Autodesk Fusion 360 part; units mm, degrees
note: some values were not read from the file. Set by a fixed rule: which sketch regions a step uses.
(part 3 of 59)
  spline S10 degree 5 poles (-22.9448, 30.3091) (-22.9448, 30.3092) (-22.945, 30.3093) (-22.9453, 30.3095) (-22.9457, 30.3098) (-22.9463, 30.3103) (-22.9469, 30.3108) (-22.9477, 30.3114) (-22.9486, 30.312) (-22.9496, 30.3127) (-22.9506, 30.3135) (-22.9518, 30.3144) (-22.953, 30.3153) (-22.9543, 30.3162) (-22.9557, 30.3172) (-22.9572, 30.3183) (-22.9588, 30.3195) (-22.9604, 30.3207) (-22.9622, 30.3219) (-22.964, 30.3232) (-22.9659, 30.3246) (-22.9679, 30.326) (-22.9699, 30.3274) (-22.9721, 30.3289) (-22.9743, 30.3305) (-22.9766, 30.3321) (-22.979, 30.3337) (-22.9814, 30.3354) (-22.984, 30.3372) (-22.9866, 30.3389) (-22.9893, 30.3408) (-22.992, 30.3427) (-22.9948, 30.3446) (-22.9978, 30.3465) (-23.0007, 30.3485) (-23.0038, 30.3506) (-23.0069, 30.3527) (-23.0101, 30.3548) (-23.0134, 30.357) (-23.0167, 30.3592) (-23.0201, 30.3614) (-23.0236, 30.3637) (-23.0271, 30.366) (-23.0308, 30.3683) (-23.0344, 30.3707) (-23.0382, 30.3731) (-23.042, 30.3756) (-23.0459, 30.3781) (-23.0499, 30.3806) (-23.0539, 30.3831) (-23.058, 30.3857) (-23.0621, 30.3883) (-23.0664, 30.391) (-23.0706, 30.3937) (-23.075, 30.3964) (-23.0794, 30.3991) (-23.0839, 30.4019) (-23.0884, 30.4047) (-23.093, 30.4075) (-23.0977, 30.4103) (-23.1024, 30.4132) (-23.1072, 30.4161) (-23.1121, 30.4191) (-23.117, 30.422) (-23.122, 30.425) (-23.127, 30.428) (-23.1321, 30.431) (-23.1373, 30.4341) (-23.1425, 30.4372) (-23.1478, 30.4403) (-23.1531, 30.4434) (-23.1585, 30.4466) (-23.164, 30.4497) (-23.1695, 30.4529) (-23.1751, 30.4562) (-23.1807, 30.4594) (-23.1864, 30.4627) (-23.1921, 30.4659) (-23.1979, 30.4692) (-23.2038, 30.4726) (-23.2097, 30.4759) (-23.2157, 30.4793) (-23.2217, 30.4826) (-23.2278, 30.486) (-23.234, 30.4895) (-23.2402, 30.4929) (-23.2464, 30.4963) (-23.2527, 30.4998) (-23.2591, 30.5033) (-23.2655, 30.5068) (-23.272, 30.5103) (-23.2785, 30.5139) (-23.2851, 30.5174) (-23.2918, 30.521) (-23.2984, 30.5246) (-23.3052, 30.5282) (-23.312, 30.5318) (-23.3188, 30.5354) (-23.3257, 30.539) (-23.3327, 30.5427) (-23.3397, 30.5464) (-23.3468, 30.5501) (-23.3539, 30.5538) (-23.361, 30.5575) (-23.3683, 30.5612) (-23.3755, 30.5649) (-23.3828, 30.5687) (-23.3902, 30.5724) (-23.3976, 30.5762) (-23.4051, 30.58) (-23.4126, 30.5838) (-23.4202, 30.5876) (-23.4278, 30.5914) (-23.4355, 30.5952) (-23.4432, 30.5991) (-23.451, 30.6029) (-23.4588, 30.6068) (-23.4666, 30.6106) (-23.4746, 30.6145) (-23.4825, 30.6184) (-23.4905, 30.6223) (-23.4986, 30.6262) (-23.5067, 30.6301) (-23.5149, 30.634) (-23.5231, 30.6379) (-23.5313, 30.6419) (-23.5396, 30.6458) (-23.548, 30.6498) (-23.5564, 30.6537) (-23.5648, 30.6577) (-23.5733, 30.6617) (-23.5818, 30.6657) (-23.5904, 30.6696) (-23.5991, 30.6736) (-23.6077, 30.6776) (-23.6165, 30.6816) (-23.6252, 30.6857) (-23.634, 30.6897) (-23.6429, 30.6937) (-23.6518, 30.6977) (-23.6607, 30.7018) (-23.6697, 30.7058) (-23.6788, 30.7098) (-23.6879, 30.7139) (-23.697, 30.7179) (-23.7062, 30.722) (-23.7154, 30.726) (-23.7247, 30.7301) (-23.734, 30.7342) (-23.7433, 30.7383) (-23.7527, 30.7423) (-23.7622, 30.7464) (-23.7716, 30.7505) (-23.7812, 30.7546) (-23.7907, 30.7587) (-23.8004, 30.7627) (-23.81, 30.7668) (-23.8197, 30.7709) (-23.8295, 30.775) (-23.8393, 30.7791) (-23.8491, 30.7832) (-23.859, 30.7873) (-23.8689, 30.7914) (-23.8788, 30.7955) (-23.8888, 30.7996) (-23.8989, 30.8038) (-23.909, 30.8079) (-23.9191, 30.812) (-23.9292, 30.8161) (-23.9395, 30.8202) (-23.9497, 30.8243) (-23.96, 30.8284) (-23.9703, 30.8325) (-23.9807, 30.8366) (-23.9911, 30.8408) (-24.0016, 30.8449) (-24.0121, 30.849) (-24.0226, 30.8531) (-24.0332, 30.8572) (-24.0438, 30.8613) (-24.0545, 30.8654) (-24.0652, 30.8695) (-24.0759, 30.8736) (-24.0867, 30.8777) (-24.0975, 30.8818) (-24.1084, 30.8859) (-24.1193, 30.89) (-24.1302, 30.8941) (-24.1412, 30.8982) (-24.1522, 30.9023) (-24.1633, 30.9064) (-24.1744, 30.9105) (-24.1855, 30.9146) (-24.1967, 30.9187) (-24.2079, 30.9228) (-24.2191, 30.9269) (-24.2304, 30.9309) (-24.2417, 30.935) (-24.2531, 30.9391) (-24.2645, 30.9431) (-24.276, 30.9472) (-24.2874, 30.9513) (-24.299, 30.9553) (-24.3105, 30.9594) (-24.3221, 30.9634) (-24.3337, 30.9675) (-24.3454, 30.9715) (-24.3571, 30.9756) (-24.3689, 30.9796) (-24.3806, 30.9836) (-24.3925, 30.9877) (-24.4043, 30.9917) (-24.4162, 30.9957) (-24.4281, 30.9997) (-24.4401, 31.0037) (-24.4521, 31.0077) (-24.4642, 31.0117) (-24.4762, 31.0157) (-24.4884, 31.0197) (-24.5005, 31.0237) (-24.5127, 31.0277) (-24.5249, 31.0316) (-24.5372, 31.0356) (-24.5495, 31.0395) (-24.5618, 31.0435) (-24.5742, 31.0475) (-24.5866, 31.0514) (-24.599, 31.0553) (-24.6115, 31.0593) (-24.624, 31.0632) (-24.6365, 31.0671) (-24.6491, 31.071) (-24.6617, 31.0749) (-24.6744, 31.0788) (-24.6871, 31.0827) (-24.6998, 31.0866) (-24.7125, 31.0905) (-24.7253, 31.0943) (-24.7382, 31.0982) (-24.751, 31.1021) (-24.7639, 31.1059) (-24.7743, 31.109) (-24.782, 31.1113) (-24.7872, 31.1128) (-24.7898, 31.1136) knots 0 0 0 0 0 0 0.00416667 0.00833333 0.0125 0.01666667 0.02083333 0.025 0.02916667 0.03333333 0.0375 0.04166667 0.04583333 0.05 0.05416667 0.05833333 0.0625 0.06666667 0.07083333 0.075 0.07916667 0.08333333 0.0875 0.09166667 0.09583333 0.1 0.10416667 0.10833333 0.1125 0.11666667 0.12083333 0.125 0.12916667 0.13333333 0.1375 0.14166667 0.14583333 0.15 0.15416667 0.15833333 0.1625 0.16666667 0.17083333 0.175 0.17916667 0.18333333 0.1875 0.19166667 0.19583333 0.2 0.20416667 0.20833333 0.2125 0.21666667 0.22083333 0.225 0.22916667 0.23333333 0.2375 0.24166667 0.24583333 0.25 0.25416667 0.25833333 0.2625 0.26666667 0.27083333 0.275 0.27916667 0.28333333 0.2875 0.29166667 0.29583333 0.3 0.30416667 0.30833333 0.3125 0.31666667 0.32083333 0.325 0.32916667 0.33333333 0.3375 0.34166667 0.34583333 0.35 0.35416667 0.35833333 0.3625 0.36666667 0.37083333 0.375 0.37916667 0.38333333 0.3875 0.39166667 0.39583333 0.4 0.40416667 0.40833333 0.4125 0.41666667 0.42083333 0.425 0.42916667 0.43333333 0.4375 0.44166667 0.44583333 0.45 0.45416667 0.45833333 0.4625 0.46666667 0.47083333 0.475 0.47916667 0.48333333 0.4875 0.49166667 0.49583333 0.5 0.50416667 0.50833333 0.5125 0.51666667 0.52083333 0.525 0.52916667 0.53333333 0.5375 0.54166667 0.54583333 0.55 0.55416667 0.55833333 0.5625 0.56666667 0.57083333 0.575 0.57916667 0.58333333 0.5875 0.59166667 0.59583333 0.6 0.60416667 0.60833333 0.6125 0.61666667 0.62083333 0.625 0.62916667 0.63333333 0.6375 0.64166667 0.64583333 0.65 0.65416667 0.65833333 0.6625 0.66666667 0.67083333 0.675 0.67916667 0.68333333 0.6875 0.69166667 0.69583333 0.7 0.70416667 0.70833333 0.7125 0.71666667 0.72083333 0.725 0.72916667 0.73333333 0.7375 0.74166667 0.74583333 0.75 0.75416667 0.75833333 0.7625 0.76666667 0.77083333 0.775 0.77916667 0.78333333 0.7875 0.79166667 0.79583333 0.8 0.80416667 0.80833333 0.8125 0.81666667 0.82083333 0.825 0.82916667 0.83333333 0.8375 0.84166667 0.84583333 0.85 0.85416667 0.85833333 0.8625 0.86666667 0.87083333 0.875 0.87916667 0.88333333 0.8875 0.89166667 0.89583333 0.9 0.90416667 0.90833333 0.9125 0.91666667 0.92083333 0.925 0.92916667 0.93333333 0.9375 0.94166667 0.94583333 0.95 0.95416667 0.95833333 0.9625 0.96666667 0.97083333 0.975 0.97916667 0.98333333 0.9875 0.99166667 0.99583333 1 1 1 1 1 1
  line L45 (-13.578, 37.8417) -> (-13.7171, 38.1012)
  line L46 (-13.7171, 38.1012) -> (-13.7175, 38.1019)
  line L47 (-2.0967, 41.1734) -> (-2.1182, 41.4671)
  spline S11 degree 5 poles (-28.5878, 7.3654) (-28.5879, 7.3653) (-28.5881, 7.3653) (-28.5884, 7.3652) (-28.5889, 7.3651) (-28.5896, 7.365) (-28.5905, 7.3648) (-28.5915, 7.3646) (-28.5925, 7.3644) (-28.5937, 7.3642) (-28.595, 7.3639) (-28.5964, 7.3637) (-28.5979, 7.3633) (-28.5995, 7.363) (-28.6012, 7.3626) (-28.603, 7.3623) (-28.6049, 7.3619) (-28.6069, 7.3614) (-28.6089, 7.361) (-28.6111, 7.3605) (-28.6134, 7.36) (-28.6158, 7.3594) (-28.6182, 7.3589) (-28.6208, 7.3583) (-28.6234, 7.3577) (-28.6262, 7.357) (-28.629, 7.3564) (-28.6319, 7.3557) (-28.6349, 7.355) (-28.6379, 7.3542) (-28.6411, 7.3535) (-28.6443, 7.3527) (-28.6477, 7.3519) (-28.6511, 7.351) (-28.6545, 7.3501) (-28.6581, 7.3492) (-28.6617, 7.3483) (-28.6655, 7.3473) (-28.6693, 7.3464) (-28.6731, 7.3454) (-28.6771, 7.3443) (-28.6811, 7.3433) (-28.6852, 7.3422) (-28.6893, 7.3411) (-28.6936, 7.3399) (-28.6979, 7.3387) (-28.7023, 7.3375) (-28.7067, 7.3363) (-28.7112, 7.3351) (-28.7158, 7.3338) (-28.7205, 7.3325) (-28.7252, 7.3311) (-28.73, 7.3298) (-28.7349, 7.3284) (-28.7398, 7.327) (-28.7448, 7.3255) (-28.7498, 7.324) (-28.7549, 7.3225) (-28.7601, 7.321) (-28.7654, 7.3194) (-28.7707, 7.3178) (-28.776, 7.3162) (-28.7815, 7.3146) (-28.7869, 7.3129) (-28.7925, 7.3112) (-28.7981, 7.3095) (-28.8038, 7.3077) (-28.8095, 7.3059) (-28.8153, 7.3041) (-28.8211, 7.3022) (-28.827, 7.3004) (-28.833, 7.2985) (-28.839, 7.2965) (-28.8451, 7.2946) (-28.8512, 7.2926) (-28.8573, 7.2906) (-28.8636, 7.2885) (-28.8699, 7.2864) (-28.8762, 7.2843) (-28.8826, 7.2822) (-28.889, 7.28) (-28.8955, 7.2778) (-28.9021, 7.2756) (-28.9087, 7.2734) (-28.9153, 7.2711) (-28.922, 7.2688) (-28.9288, 7.2664) (-28.9356, 7.2641) (-28.9424, 7.2617) (-28.9493, 7.2592) (-28.9563, 7.2568) (-28.9633, 7.2543) (-28.9703, 7.2518) (-28.9774, 7.2492) (-28.9846, 7.2467) (-28.9918, 7.2441) (-28.999, 7.2414) (-29.0063, 7.2388) (-29.0136, 7.2361) (-29.021, 7.2334) (-29.0284, 7.2306) (-29.0358, 7.2278) (-29.0433, 7.225) (-29.0509, 7.2222) (-29.0585, 7.2193) (-29.0661, 7.2164) (-29.0738, 7.2135) (-29.0815, 7.2105) (-29.0893, 7.2075) (-29.0971, 7.2045) (-29.105, 7.2014) (-29.1129, 7.1984) (-29.1208, 7.1953) (-29.1288, 7.1921) (-29.1368, 7.1889) (-29.1448, 7.1857) (-29.1529, 7.1825) (-29.1611, 7.1793) (-29.1692, 7.176) (-29.1775, 7.1727) (-29.1857, 7.1693) (-29.194, 7.1659) (-29.2023, 7.1625) (-29.2107, 7.1591) (-29.2191, 7.1556) (-29.2276, 7.1521) (-29.2361, 7.1486) (-29.2446, 7.145) (-29.2531, 7.1414) (-29.2617, 7.1378) (-29.2704, 7.1342) (-29.279, 7.1305) (-29.2878, 7.1268) (-29.2965, 7.123) (-29.3053, 7.1193) (-29.3141, 7.1154) (-29.3229, 7.1116) (-29.3318, 7.1078) (-29.3407, 7.1039) (-29.3497, 7.0999) (-29.3587, 7.096) (-29.3677, 7.092) (-29.3767, 7.088) (-29.3858, 7.0839) (-29.395, 7.0799) (-29.4041, 7.0758) (-29.4133, 7.0716) (-29.4225, 7.0675) (-29.4318, 7.0633) (-29.441, 7.059) (-29.4504, 7.0548) (-29.4597, 7.0505) (-29.4691, 7.0462) (-29.4785, 7.0418) (-29.4879, 7.0375) (-29.4974, 7.033) (-29.5069, 7.0286) (-29.5165, 7.0241) (-29.526, 7.0196) (-29.5356, 7.0151) (-29.5452, 7.0105) (-29.5549, 7.006) (-29.5646, 7.0013) (-29.5743, 6.9967) (-29.584, 6.992) (-29.5938, 6.9873) (-29.6036, 6.9825) (-29.6134, 6.9778) (-29.6233, 6.973) (-29.6332, 6.9681) (-29.6431, 6.9633) (-29.653, 6.9584) (-29.663, 6.9534) (-29.673, 6.9485) (-29.683, 6.9435) (-29.6931, 6.9385) (-29.7032, 6.9334) (-29.7133, 6.9283) (-29.7234, 6.9232) (-29.7336, 6.9181) (-29.7437, 6.9129) (-29.754, 6.9077) (-29.7642, 6.9025) (-29.7745, 6.8972) (-29.7847, 6.8919) (-29.7951, 6.8866) (-29.8054, 6.8812) (-29.8158, 6.8758) (-29.8262, 6.8704) (-29.8366, 6.865) (-29.847, 6.8595) (-29.8575, 6.854) (-29.868, 6.8485) (-29.8785, 6.8429) (-29.889, 6.8373) (-29.8996, 6.8317) (-29.9102, 6.826) (-29.9208, 6.8203) (-29.9314, 6.8146) (-29.9421, 6.8088) (-29.9527, 6.803) (-29.9634, 6.7972) (-29.9742, 6.7914) (-29.9849, 6.7855) (-29.9957, 6.7796) (-30.0065, 6.7737) (-30.0173, 6.7677) (-30.0281, 6.7617) (-30.039, 6.7557) (-30.0499, 6.7496) (-30.0608, 6.7435) (-30.0717, 6.7374) (-30.0826, 6.7312) (-30.0936, 6.7251) (-30.1046, 6.7189) (-30.1156, 6.7126) (-30.1266, 6.7063) (-30.1377, 6.7) (-30.1487, 6.6937) (-30.1598, 6.6873) (-30.1709, 6.6809) (-30.1821, 6.6745) (-30.1932, 6.6681) (-30.2044, 6.6616) (-30.2156, 6.6551) (-30.2268, 6.6485) (-30.238, 6.6419) (-30.2492, 6.6353) (-30.2605, 6.6287) (-30.2718, 6.622) (-30.2831, 6.6153) (-30.2944, 6.6086) (-30.3058, 6.6018) (-30.3171, 6.595) (-30.3285, 6.5882) (-30.3399, 6.5813) (-30.3513, 6.5745) (-30.3628, 6.5675) (-30.3742, 6.5606) (-30.3857, 6.5536) (-30.3972, 6.5466) (-30.4064, 6.541) (-30.4133, 6.5367) (-30.4179, 6.5339) (-30.4202, 6.5325) knots 0 0 0 0 0 0 0.00416667 0.00833333 0.0125 0.01666667 0.02083333 0.025 0.02916667 0.03333333 0.0375 0.04166667 0.04583333 0.05 0.05416667 0.05833333 0.0625 0.06666667 0.07083333 0.075 0.07916667 0.08333333 0.0875 0.09166667 0.09583333 0.1 0.10416667 0.10833333 0.1125 0.11666667 0.12083333 0.125 0.12916667 0.13333333 0.1375 0.14166667 0.14583333 0.15 0.15416667 0.15833333 0.1625 0.16666667 0.17083333 0.175 0.17916667 0.18333333 0.1875 0.19166667 0.19583333 0.2 0.20416667 0.20833333 0.2125 0.21666667 0.22083333 0.225 0.22916667 0.23333333 0.2375 0.24166667 0.24583333 0.25 0.25416667 0.25833333 0.2625 0.26666667 0.27083333 0.275 0.27916667 0.28333333 0.2875 0.29166667 0.29583333 0.3 0.30416667 0.30833333 0.3125 0.31666667 0.32083333 0.325 0.32916667 0.33333333 0.3375 0.34166667 0.34583333 0.35 0.35416667 0.35833333 0.3625 0.36666667 0.37083333 0.375 0.37916667 0.38333333 0.3875 0.39166667 0.39583333 0.4 0.40416667 0.40833333 0.4125 0.41666667 0.42083333 0.425 0.42916667 0.43333333 0.4375 0.44166667 0.44583333 0.45 0.45416667 0.45833333 0.4625 0.46666667 0.47083333 0.475 0.47916667 0.48333333 0.4875 0.49166667 0.49583333 0.5 0.50416667 0.50833333 0.5125 0.51666667 0.52083333 0.525 0.52916667 0.53333333 0.5375 0.54166667 0.54583333 0.55 0.55416667 0.55833333 0.5625 0.56666667 0.57083333 0.575 0.57916667 0.58333333 0.5875 0.59166667 0.59583333 0.6 0.60416667 0.60833333 0.6125 0.61666667 0.62083333 0.625 0.62916667 0.63333333 0.6375 0.64166667 0.64583333 0.65 0.65416667 0.65833333 0.6625 0.66666667 0.67083333 0.675 0.67916667 0.68333333 0.6875 0.69166667 0.69583333 0.7 0.70416667 0.70833333 0.7125 0.71666667 0.72083333 0.725 0.72916667 0.73333333 0.7375 0.74166667 0.74583333 0.75 0.75416667 0.75833333 0.7625 0.76666667 0.77083333 0.775 0.77916667 0.78333333 0.7875 0.79166667 0.79583333 0.8 0.80416667 0.80833333 0.8125 0.81666667 0.82083333 0.825 0.82916667 0.83333333 0.8375 0.84166667 0.84583333 0.85 0.85416667 0.85833333 0.8625 0.86666667 0.87083333 0.875 0.87916667 0.88333333 0.8875 0.89166667 0.89583333 0.9 0.90416667 0.90833333 0.9125 0.91666667 0.92083333 0.925 0.92916667 0.93333333 0.9375 0.94166667 0.94583333 0.95 0.95416667 0.95833333 0.9625 0.96666667 0.97083333 0.975 0.97916667 0.98333333 0.9875 0.99166667 0.99583333 1 1 1 1 1 1
  line L48 (-25.6019, 26.2175) -> (-25.6012, 26.2171)
  spline S12 degree 5 poles (-27.0873, 27.5758) (-27.0855, 27.5737) (-27.082, 27.5696) (-27.0767, 27.5635) (-27.0697, 27.5553) (-27.061, 27.545) (-27.0522, 27.5349) (-27.0435, 27.5247) (-27.0347, 27.5146) (-27.026, 27.5045) (-27.0173, 27.4945) (-27.0086, 27.4845) (-26.9999, 27.4745) (-26.9912, 27.4646) (-26.9825, 27.4547) (-26.9738, 27.4448) (-26.9651, 27.435) (-26.9565, 27.4252) (-26.9478, 27.4154) (-26.9392, 27.4057) (-26.9305, 27.396) (-26.9219, 27.3863) (-26.9133, 27.3767) (-26.9047, 27.3671) (-26.8961, 27.3576) (-26.8875, 27.3481) (-26.8789, 27.3386) (-26.8703, 27.3291) (-26.8618, 27.3197) (-26.8532, 27.3104) (-26.8447, 27.301) (-26.8361, 27.2917) (-26.8276, 27.2824) (-26.8191, 27.2732) (-26.8106, 27.264) (-26.8021, 27.2549) (-26.7937, 27.2457) (-26.7852, 27.2366) (-26.7767, 27.2276) (-26.7683, 27.2186) (-26.7599, 27.2096) (-26.7515, 27.2006) (-26.7431, 27.1917) (-26.7347, 27.1829) (-26.7263, 27.174) (-26.7179, 27.1652) (-26.7096, 27.1565) (-26.7012, 27.1477) (-26.6929, 27.139) (-26.6846, 27.1304) (-26.6763, 27.1218) (-26.668, 27.1132) (-26.6597, 27.1046) (-26.6514, 27.0961) (-26.6432, 27.0877) (-26.635, 27.0792) (-26.6267, 27.0708) (-26.6185, 27.0625) (-26.6103, 27.0541) (-26.6022, 27.0459) (-26.594, 27.0376) (-26.5858, 27.0294) (-26.5777, 27.0212) (-26.5696, 27.0131) (-26.5615, 27.005) (-26.5534, 26.9969) (-26.5453, 26.9889) (-26.5373, 26.9809) (-26.5292, 26.9729) (-26.5212, 26.965) (-26.5132, 26.9571) (-26.5052, 26.9493) (-26.4972, 26.9415) (-26.4893, 26.9337) (-26.4813, 26.926) (-26.4734, 26.9183) (-26.4655, 26.9106) (-26.4576, 26.903) (-26.4497, 26.8954) (-26.4419, 26.8879) (-26.434, 26.8804) (-26.4262, 26.8729) (-26.4184, 26.8655) (-26.4106, 26.8581) (-26.4029, 26.8508) (-26.3951, 26.8435) (-26.3874, 26.8362) (-26.3797, 26.8289) (-26.372, 26.8217) (-26.3643, 26.8146) (-26.3567, 26.8075) (-26.3491, 26.8004) (-26.3414, 26.7933) (-26.3339, 26.7863) (-26.3263, 26.7794) (-26.3188, 26.7724) (-26.3112, 26.7656) (-26.3037, 26.7587) (-26.2962, 26.7519) (-26.2888, 26.7451) (-26.2813, 26.7384) (-26.2739, 26.7317) (-26.2665, 26.725) (-26.2592, 26.7184) (-26.2518, 26.7119) (-26.2445, 26.7053) (-26.2372, 26.6988) (-26.2299, 26.6924) (-26.2227, 26.6859) (-26.2154, 26.6796) (-26.2082, 26.6732) (-26.201, 26.6669) (-26.1939, 26.6607) (-26.1868, 26.6544) (-26.1796, 26.6483) (-26.1726, 26.6421) (-26.1655, 26.636) (-26.1585, 26.63) (-26.1515, 26.6239) (-26.1445, 26.618) (-26.1375, 26.612) (-26.1306, 26.6061) (-26.1237, 26.6003) (-26.1168, 26.5945) (-26.11, 26.5887) (-26.1032, 26.5829) (-26.0964, 26.5772) (-26.0896, 26.5716) (-26.0829, 26.566) (-26.0762, 26.5604) (-26.0695, 26.5549) (-26.0629, 26.5494) (-26.0563, 26.5439) (-26.0497, 26.5385) (-26.0431, 26.5332) (-26.0366, 26.5278) (-26.0301, 26.5225) (-26.0236, 26.5173) (-26.0172, 26.5121) (-26.0108, 26.5069) (-26.0044, 26.5018) (-25.9981, 26.4967) (-25.9918, 26.4917) (-25.9855, 26.4867) (-25.9793, 26.4818) (-25.9731, 26.4769) (-25.9669, 26.472) (-25.9608, 26.4672) (-25.9547, 26.4624) (-25.9486, 26.4576) (-25.9426, 26.4529) (-25.9366, 26.4483) (-25.9306, 26.4437) (-25.9247, 26.4391) (-25.9188, 26.4346) (-25.913, 26.4301) (-25.9072, 26.4257) (-25.9014, 26.4213) (-25.8957, 26.4169) (-25.89, 26.4126) (-25.8843, 26.4083) (-25.8787, 26.4041) (-25.8731, 26.3999) (-25.8676, 26.3958) (-25.8621, 26.3917) (-25.8566, 26.3876) (-25.8512, 26.3836) (-25.8458, 26.3797) (-25.8405, 26.3758) (-25.8352, 26.3719) (-25.8299, 26.3681) (-25.8247, 26.3643) (-25.8195, 26.3605) (-25.8144, 26.3568) (-25.8093, 26.3532) (-25.8043, 26.3496) (-25.7993, 26.346) (-25.7944, 26.3425) (-25.7895, 26.339) (-25.7847, 26.3356) (-25.7799, 26.3322) (-25.7751, 26.3289) (-25.7704, 26.3256) (-25.7658, 26.3224) (-25.7612, 26.3192) (-25.7566, 26.316) (-25.7521, 26.3129) (-25.7476, 26.3098) (-25.7432, 26.3068) (-25.7389, 26.3039) (-25.7346, 26.3009) (-25.7304, 26.2981) (-25.7262, 26.2952) (-25.722, 26.2925) (-25.718, 26.2897) (-25.7139, 26.287) (-25.71, 26.2844) (-25.706, 26.2818) (-25.7022, 26.2793) (-25.6984, 26.2768) (-25.6947, 26.2743) (-25.691, 26.2719) (-25.6874, 26.2696) (-25.6838, 26.2673) (-25.6803, 26.265) (-25.6769, 26.2628) (-25.6735, 26.2607) (-25.6702, 26.2586) (-25.667, 26.2565) (-25.6638, 26.2545) (-25.6607, 26.2526) (-25.6577, 26.2506) (-25.6547, 26.2488) (-25.6518, 26.247) (-25.6489, 26.2452) (-25.6462, 26.2435) (-25.6435, 26.2419) (-25.6409, 26.2403) (-25.6383, 26.2387) (-25.6358, 26.2372) (-25.6334, 26.2358) (-25.6311, 26.2344) (-25.6289, 26.233) (-25.6267, 26.2317) (-25.6246, 26.2305) (-25.6226, 26.2293) (-25.6207, 26.2282) (-25.6188, 26.2271) (-25.6171, 26.2261) (-25.6154, 26.2251) (-25.6138, 26.2242) (-25.6123, 26.2233) (-25.6109, 26.2225) (-25.6096, 26.2217) (-25.6083, 26.221) (-25.6072, 26.2204) (-25.6061, 26.2198) (-25.6052, 26.2193) (-25.6043, 26.2188) (-25.6036, 26.2184) (-25.6029, 26.218) (-25.6025, 26.2178) (-25.6022, 26.2176) (-25.602, 26.2175) (-25.6019, 26.2175) knots -1 -1 -1 -1 -1 -1 -0.99583333 -0.99166667 -0.9875 -0.98333333 -0.97916667 -0.975 -0.97083333 -0.96666667 -0.9625 -0.95833333 -0.95416667 -0.95 -0.94583333 -0.94166667 -0.9375 -0.93333333 -0.92916667 -0.925 -0.92083333 -0.91666667 -0.9125 -0.90833333 -0.90416667 -0.9 -0.89583333 -0.89166667 -0.8875 -0.88333333 -0.87916667 -0.875 -0.87083333 -0.86666667 -0.8625 -0.85833333 -0.85416667 -0.85 -0.84583333 -0.84166667 -0.8375 -0.83333333 -0.82916667 -0.825 -0.82083333 -0.81666667 -0.8125 -0.80833333 -0.80416667 -0.8 -0.79583333 -0.79166667 -0.7875 -0.78333333 -0.77916667 -0.775 -0.77083333 -0.76666667 -0.7625 -0.75833333 -0.75416667 -0.75 -0.74583333 -0.74166667 -0.7375 -0.73333333 -0.72916667 -0.725 -0.72083333 -0.71666667 -0.7125 -0.70833333 -0.70416667 -0.7 -0.69583333 -0.69166667 -0.6875 -0.68333333 -0.67916667 -0.675 -0.67083333 -0.66666667 -0.6625 -0.65833333 -0.65416667 -0.65 -0.64583333 -0.64166667 -0.6375 -0.63333333 -0.62916667 -0.625 -0.62083333 -0.61666667 -0.6125 -0.60833333 -0.60416667 -0.6 -0.59583333 -0.59166667 -0.5875 -0.58333333 -0.57916667 -0.575 -0.57083333 -0.56666667 -0.5625 -0.55833333 -0.55416667 -0.55 -0.54583333 -0.54166667 -0.5375 -0.53333333 -0.52916667 -0.525 -0.52083333 -0.51666667 -0.5125 -0.50833333 -0.50416667 -0.5 -0.49583333 -0.49166667 -0.4875 -0.48333333 -0.47916667 -0.475 -0.47083333 -0.46666667 -0.4625 -0.45833333 -0.45416667 -0.45 -0.44583333 -0.44166667 -0.4375 -0.43333333 -0.42916667 -0.425 -0.42083333 -0.41666667 -0.4125 -0.40833333 -0.40416667 -0.4 -0.39583333 -0.39166667 -0.3875 -0.38333333 -0.37916667 -0.375 -0.37083333 -0.36666667 -0.3625 -0.35833333 -0.35416667 -0.35 -0.34583333 -0.34166667 -0.3375 -0.33333333 -0.32916667 -0.325 -0.32083333 -0.31666667 -0.3125 -0.30833333 -0.30416667 -0.3 -0.29583333 -0.29166667 -0.2875 -0.28333333 -0.27916667 -0.275 -0.27083333 -0.26666667 -0.2625 -0.25833333 -0.25416667 -0.25 -0.24583333 -0.24166667 -0.2375 -0.23333333 -0.22916667 -0.225 -0.22083333 -0.21666667 -0.2125 -0.20833333 -0.20416667 -0.2 -0.19583333 -0.19166667 -0.1875 -0.18333333 -0.17916667 -0.175 -0.17083333 -0.16666667 -0.1625 -0.15833333 -0.15416667 -0.15 -0.14583333 -0.14166667 -0.1375 -0.13333333 -0.12916667 -0.125 -0.12083333 -0.11666667 -0.1125 -0.10833333 -0.10416667 -0.1 -0.09583333 -0.09166667 -0.0875 -0.08333333 -0.07916667 -0.075 -0.07083333 -0.06666667 -0.0625 -0.05833333 -0.05416667 -0.05 -0.04583333 -0.04166667 -0.0375 -0.03333333 -0.02916667 -0.025 -0.02083333 -0.01666667 -0.0125 -0.00833333 -0.00416667 0 0 0 0 0 0
  spline S13 degree 5 poles (-24.6806, 27.8132) (-24.6807, 27.8132) (-24.6809, 27.8133) (-24.6812, 27.8135) (-24.6816, 27.8138) (-24.6822, 27.8142) (-24.683, 27.8146) (-24.6838, 27.8151) (-24.6848, 27.8157) (-24.6858, 27.8163) (-24.6869, 27.8169) (-24.6881, 27.8177) (-24.6895, 27.8184) (-24.6909, 27.8193) (-24.6924, 27.8201) (-24.694, 27.821) (-24.6956, 27.822) (-24.6974, 27.823) (-24.6993, 27.8241) (-24.7012, 27.8252) (-24.7033, 27.8263) (-24.7054, 27.8275) (-24.7076, 27.8287) (-24.7099, 27.83) (-24.7122, 27.8313) (-24.7147, 27.8327) (-24.7172, 27.8341) (-24.7198, 27.8355) (-24.7225, 27.837) (-24.7253, 27.8385) (-24.7282, 27.84) (-24.7311, 27.8416) (-24.7341, 27.8432) (-24.7372, 27.8449) (-24.7404, 27.8465) (-24.7437, 27.8482) (-24.747, 27.85) (-24.7504, 27.8518) (-24.7539, 27.8536) (-24.7574, 27.8554) (-24.761, 27.8573) (-24.7647, 27.8592) (-24.7685, 27.8611) (-24.7723, 27.8631) (-24.7763, 27.8651) (-24.7802, 27.8671) (-24.7843, 27.8691) (-24.7884, 27.8712) (-24.7926, 27.8733) (-24.7969, 27.8754) (-24.8012, 27.8775) (-24.8056, 27.8797) (-24.8101, 27.8819) (-24.8147, 27.8841) (-24.8193, 27.8863) (-24.8239, 27.8886) (-24.8287, 27.8909) (-24.8335, 27.8932) (-24.8384, 27.8955) (-24.8433, 27.8979) (-24.8483, 27.9002) (-24.8534, 27.9026) (-24.8585, 27.905) (-24.8637, 27.9075) (-24.869, 27.9099) (-24.8743, 27.9124) (-24.8797, 27.9149) (-24.8852, 27.9174) (-24.8907, 27.9199) (-24.8962, 27.9224) (-24.9019, 27.925) (-24.9076, 27.9275) (-24.9133, 27.9301) (-24.9192, 27.9327) (-24.925, 27.9353) (-24.931, 27.938) (-24.937, 27.9406) (-24.943, 27.9433) (-24.9492, 27.946) (-24.9553, 27.9486) (-24.9616, 27.9514) (-24.9679, 27.9541) (-24.9742, 27.9568) (-24.9806, 27.9595) (-24.9871, 27.9623) (-24.9936, 27.9651) (-25.0002, 27.9678) (-25.0069, 27.9706) (-25.0136, 27.9734) (-25.0203, 27.9762) (-25.0271, 27.9791) (-25.034, 27.9819) (-25.0409, 27.9848) (-25.0479, 27.9876) (-25.0549, 27.9905) (-25.062, 27.9933) (-25.0691, 27.9962) (-25.0763, 27.9991) (-25.0836, 28.002) (-25.0909, 28.0049) (-25.0982, 28.0078) (-25.1056, 28.0108) (-25.1131, 28.0137) (-25.1206, 28.0166) (-25.1282, 28.0196) (-25.1358, 28.0226) (-25.1434, 28.0255) (-25.1512, 28.0285) (-25.1589, 28.0315) (-25.1668, 28.0344) (-25.1746, 28.0374) (-25.1826, 28.0404) (-25.1905, 28.0434) (-25.1986, 28.0464) (-25.2066, 28.0494) (-25.2148, 28.0524) (-25.2229, 28.0555) (-25.2312, 28.0585) (-25.2394, 28.0615) (-25.2478, 28.0645) (-25.2562, 28.0676) (-25.2646, 28.0706) (-25.2731, 28.0737) (-25.2816, 28.0767) (-25.2901, 28.0798) (-25.2988, 28.0828) (-25.3074, 28.0859) (-25.3161, 28.0889) (-25.3249, 28.092) (-25.3337, 28.095) (-25.3426, 28.0981) (-25.3515, 28.1012) (-25.3604, 28.1042) (-25.3694, 28.1073) (-25.3785, 28.1104) (-25.3876, 28.1134) (-25.3967, 28.1165) (-25.4059, 28.1196) (-25.4151, 28.1227) (-25.4244, 28.1257) (-25.4337, 28.1288) (-25.4431, 28.1319) (-25.4525, 28.135) (-25.462, 28.138) (-25.4715, 28.1411) (-25.481, 28.1442) (-25.4906, 28.1473) (-25.5003, 28.1503) (-25.5099, 28.1534) (-25.5197, 28.1565) (-25.5294, 28.1596) (-25.5393, 28.1626) (-25.5491, 28.1657) (-25.559, 28.1688) (-25.569, 28.1718) (-25.579, 28.1749) (-25.589, 28.1779) (-25.5991, 28.181) (-25.6092, 28.1841) (-25.6194, 28.1871) (-25.6296, 28.1902) (-25.6398, 28.1932) (-25.6501, 28.1963) (-25.6604, 28.1993) (-25.6708, 28.2023) (-25.6812, 28.2054) (-25.6917, 28.2084) (-25.7022, 28.2114) (-25.7127, 28.2145) (-25.7233, 28.2175) (-25.7339, 28.2205) (-25.7446, 28.2235) (-25.7553, 28.2265) (-25.766, 28.2295) (-25.7768, 28.2325) (-25.7877, 28.2355) (-25.7985, 28.2385) (-25.8094, 28.2415) (-25.8204, 28.2445) (-25.8314, 28.2475) (-25.8424, 28.2504) (-25.8535, 28.2534) (-25.8646, 28.2564) (-25.8757, 28.2593) (-25.8869, 28.2623) (-25.8982, 28.2652) (-25.9094, 28.2682) (-25.9207, 28.2711) (-25.9321, 28.274) (-25.9435, 28.2769) (-25.9549, 28.2798) (-25.9663, 28.2828) (-25.9778, 28.2857) (-25.9894, 28.2886) (-26.001, 28.2914) (-26.0126, 28.2943) (-26.0242, 28.2972) (-26.0359, 28.3001) (-26.0477, 28.3029) (-26.0594, 28.3058) (-26.0712, 28.3086) (-26.0831, 28.3115) (-26.095, 28.3143) (-26.1069, 28.3171) (-26.1188, 28.3199) (-26.1308, 28.3227) (-26.1428, 28.3255) (-26.1549, 28.3283) (-26.167, 28.3311) (-26.1792, 28.3339) (-26.1913, 28.3367) (-26.2035, 28.3394) (-26.2158, 28.3422) (-26.2281, 28.3449) (-26.2404, 28.3477) (-26.2528, 28.3504) (-26.2651, 28.3531) (-26.2776, 28.3558) (-26.29, 28.3585) (-26.3025, 28.3612) (-26.3151, 28.3639) (-26.3276, 28.3666) (-26.3403, 28.3692) (-26.3529, 28.3719) (-26.3656, 28.3745) (-26.3783, 28.3771) (-26.391, 28.3798) (-26.4038, 28.3824) (-26.4166, 28.385) (-26.4295, 28.3876) (-26.4424, 28.3902) (-26.4553, 28.3927) (-26.4682, 28.3953) (-26.4812, 28.3979) (-26.4943, 28.4004) (-26.5073, 28.4029) (-26.5204, 28.4055) (-26.5335, 28.408) (-26.5467, 28.4105) (-26.5599, 28.413) (-26.5731, 28.4154) (-26.5837, 28.4174) (-26.5917, 28.4189) (-26.597, 28.4199) (-26.5997, 28.4204) knots 0 0 0 0 0 0 0.00416667 0.00833333 0.0125 0.01666667 0.02083333 0.025 0.02916667 0.03333333 0.0375 0.04166667 0.04583333 0.05 0.05416667 0.05833333 0.0625 0.06666667 0.07083333 0.075 0.07916667 0.08333333 0.0875 0.09166667 0.09583333 0.1 0.10416667 0.10833333 0.1125 0.11666667 0.12083333 0.125 0.12916667 0.13333333 0.1375 0.14166667 0.14583333 0.15 0.15416667 0.15833333 0.1625 0.16666667 0.17083333 0.175 0.17916667 0.18333333 0.1875 0.19166667 0.19583333 0.2 0.20416667 0.20833333 0.2125 0.21666667 0.22083333 0.225 0.22916667 0.23333333 0.2375 0.24166667 0.24583333 0.25 0.25416667 0.25833333 0.2625 0.26666667 0.27083333 0.275 0.27916667 0.28333333 0.2875 0.29166667 0.29583333 0.3 0.30416667 0.30833333 0.3125 0.31666667 0.32083333 0.325 0.32916667 0.33333333 0.3375 0.34166667 0.34583333 0.35 0.35416667 0.35833333 0.3625 0.36666667 0.37083333 0.375 0.37916667 0.38333333 0.3875 0.39166667 0.39583333 0.4 0.40416667 0.40833333 0.4125 0.41666667 0.42083333 0.425 0.42916667 0.43333333 0.4375 0.44166667 0.44583333 0.45 0.45416667 0.45833333 0.4625 0.46666667 0.47083333 0.475 0.47916667 0.48333333 0.4875 0.49166667 0.49583333 0.5 0.50416667 0.50833333 0.5125 0.51666667 0.52083333 0.525 0.52916667 0.53333333 0.5375 0.54166667 0.54583333 0.55 0.55416667 0.55833333 0.5625 0.56666667 0.57083333 0.575 0.57916667 0.58333333 0.5875 0.59166667 0.59583333 0.6 0.60416667 0.60833333 0.6125 0.61666667 0.62083333 0.625 0.62916667 0.63333333 0.6375 0.64166667 0.64583333 0.65 0.65416667 0.65833333 0.6625 0.66666667 0.67083333 0.675 0.67916667 0.68333333 0.6875 0.69166667 0.69583333 0.7 0.70416667 0.70833333 0.7125 0.71666667 0.72083333 0.725 0.72916667 0.73333333 0.7375 0.74166667 0.74583333 0.75 0.75416667 0.75833333 0.7625 0.76666667 0.77083333 0.775 0.77916667 0.78333333 0.7875 0.79166667 0.79583333 0.8 0.80416667 0.80833333 0.8125 0.81666667 0.82083333 0.825 0.82916667 0.83333333 0.8375 0.84166667 0.84583333 0.85 0.85416667 0.85833333 0.8625 0.86666667 0.87083333 0.875 0.87916667 0.88333333 0.8875 0.89166667 0.89583333 0.9 0.90416667 0.90833333 0.9125 0.91666667 0.92083333 0.925 0.92916667 0.93333333 0.9375 0.94166667 0.94583333 0.95 0.95416667 0.95833333 0.9625 0.96666667 0.97083333 0.975 0.97916667 0.98333333 0.9875 0.99166667 0.99583333 1 1 1 1 1 1
  arc A24 (-23.7836, 28.6526) -> (-24.4297, 27.6575) centre (0, 12.5) ccw
  line L49 (-24.4297, 27.6575) -> (-24.6799, 27.8128)
  line L50 (-24.6799, 27.8128) -> (-24.6806, 27.8132)
  line L51 (-0.9213, 41.5307) -> (-0.9213, 41.5298)
  line L52 (-2.1182, 41.4671) -> (-2.1183, 41.4679)
  line L53 (-12.6491, 38.6453) -> (-12.5209, 38.3803)
  line L54 (-25.6012, 26.2171) -> (-25.3417, 26.078)
  line L55 (-24.0271, 28.818) -> (-23.7836, 28.6526)
  line L56 (-12.6495, 38.6461) -> (-12.6491, 38.6453)
  arc A25 (-24.7898, 31.1136) -> (-25.363, 30.3246) centre (0, 12.5) ccw
  line L57 (-24.0278, 28.8184) -> (-24.0271, 28.818)
  line L58 (-26.1453, 25.1491) -> (-26.1461, 25.1495)
  line L59 (-25.8803, 25.0209) -> (-26.1453, 25.1491)
  spline S14 degree 5 poles (-25.363, 30.3246) (-25.3615, 30.3224) (-25.3584, 30.3179) (-25.3539, 30.3112) (-25.3477, 30.3023) (-25.3401, 30.2913) (-25.3325, 30.2802) (-25.3248, 30.2692) (-25.3172, 30.2583) (-25.3096, 30.2473) (-25.3019, 30.2364) (-25.2943, 30.2256) (-25.2867, 30.2147) (-25.2791, 30.2039) (-25.2715, 30.1932) (-25.2639, 30.1825) (-25.2563, 30.1718) (-25.2487, 30.1611) (-25.2411, 30.1505) (-25.2335, 30.1399) (-25.2259, 30.1294) (-25.2184, 30.1189) (-25.2108, 30.1084) (-25.2032, 30.098) (-25.1957, 30.0876) (-25.1881, 30.0772) (-25.1806, 30.0669) (-25.1731, 30.0566) (-25.1655, 30.0464) (-25.158, 30.0361) (-25.1505, 30.026) (-25.143, 30.0158) (-25.1355, 30.0057) (-25.128, 29.9956) (-25.1205, 29.9856) (-25.113, 29.9756) (-25.1055, 29.9657) (-25.0981, 29.9557) (-25.0906, 29.9458) (-25.0832, 29.936) (-25.0757, 29.9262) (-25.0683, 29.9164) (-25.0609, 29.9067) (-25.0534, 29.897) (-25.046, 29.8873) (-25.0386, 29.8777) (-25.0312, 29.8681) (-25.0238, 29.8585) (-25.0165, 29.849) (-25.0091, 29.8395) (-25.0017, 29.8301) (-24.9944, 29.8207) (-24.9871, 29.8113) (-24.9797, 29.802) (-24.9724, 29.7927) (-24.9651, 29.7835) (-24.9578, 29.7743) (-24.9505, 29.7651) (-24.9432, 29.7559) (-24.936, 29.7469) (-24.9287, 29.7378) (-24.9215, 29.7288) (-24.9142, 29.7198) (-24.907, 29.7108) (-24.8998, 29.7019) (-24.8926, 29.6931) (-24.8854, 29.6842) (-24.8782, 29.6754) (-24.8711, 29.6667) (-24.8639, 29.658) (-24.8568, 29.6493) (-24.8496, 29.6407) (-24.8425, 29.6321) (-24.8354, 29.6235) (-24.8283, 29.615) (-24.8212, 29.6065) (-24.8142, 29.5981) (-24.8071, 29.5897) (-24.8001, 29.5813) (-24.7931, 29.573) (-24.7861, 29.5647) (-24.7791, 29.5565) (-24.7721, 29.5483) (-24.7651, 29.5401) (-24.7582, 29.532) (-24.7512, 29.5239) (-24.7443, 29.5159) (-24.7374, 29.5079) (-24.7305, 29.4999) (-24.7236, 29.492) (-24.7168, 29.4841) (-24.7099, 29.4763) (-24.7031, 29.4685) (-24.6963, 29.4607) (-24.6895, 29.453) (-24.6827, 29.4453) (-24.6759, 29.4377) (-24.6692, 29.4301) (-24.6625, 29.4225) (-24.6558, 29.415) (-24.6491, 29.4075) (-24.6424, 29.4001) (-24.6357, 29.3927) (-24.6291, 29.3854) (-24.6225, 29.3781) (-24.6159, 29.3708) (-24.6093, 29.3636) (-24.6027, 29.3564) (-24.5962, 29.3492) (-24.5897, 29.3421) (-24.5831, 29.3351) (-24.5767, 29.3281) (-24.5702, 29.3211) (-24.5638, 29.3142) (-24.5573, 29.3073) (-24.5509, 29.3004) (-24.5446, 29.2936) (-24.5382, 29.2869) (-24.5319, 29.2801) (-24.5255, 29.2735) (-24.5192, 29.2668) (-24.513, 29.2602) (-24.5067, 29.2537) (-24.5005, 29.2472) (-24.4943, 29.2407) (-24.4881, 29.2343) (-24.482, 29.2279) (-24.4758, 29.2216) (-24.4697, 29.2153) (-24.4636, 29.2091) (-24.4576, 29.2029) (-24.4515, 29.1967) (-24.4455, 29.1906) (-24.4395, 29.1845) (-24.4336, 29.1785) (-24.4277, 29.1725) (-24.4218, 29.1666) (-24.4159, 29.1607) (-24.41, 29.1549) (-24.4042, 29.1491) (-24.3984, 29.1433) (-24.3926, 29.1376) (-24.3869, 29.1319) (-24.3812, 29.1263) (-24.3755, 29.1207) (-24.3698, 29.1152) (-24.3642, 29.1097) (-24.3586, 29.1043) (-24.353, 29.0989) (-24.3475, 29.0935) (-24.342, 29.0882) (-24.3365, 29.083) (-24.3311, 29.0778) (-24.3257, 29.0726) (-24.3203, 29.0675) (-24.3149, 29.0624) (-24.3096, 29.0574) (-24.3043, 29.0524) (-24.2991, 29.0475) (-24.2939, 29.0426) (-24.2887, 29.0378) (-24.2835, 29.033) (-24.2784, 29.0282) (-24.2733, 29.0236) (-24.2683, 29.0189) (-24.2633, 29.0143) (-24.2583, 29.0098) (-24.2534, 29.0053) (-24.2485, 29.0008) (-24.2436, 28.9964) (-24.2388, 28.992) (-24.234, 28.9877) (-24.2293, 28.9835) (-24.2246, 28.9793) (-24.2199, 28.9751) (-24.2153, 28.971) (-24.2107, 28.9669) (-24.2062, 28.9629) (-24.2017, 28.959) (-24.1972, 28.955) (-24.1928, 28.9512) (-24.1884, 28.9474) (-24.1841, 28.9436) (-24.1798, 28.9399) (-24.1755, 28.9362) (-24.1713, 28.9326) (-24.1672, 28.9291) (-24.1631, 28.9256) (-24.159, 28.9221) (-24.155, 28.9187) (-24.151, 28.9153) (-24.1471, 28.912) (-24.1432, 28.9088) (-24.1394, 28.9056) (-24.1356, 28.9024) (-24.1319, 28.8994) (-24.1283, 28.8963) (-24.1246, 28.8933) (-24.1211, 28.8904) (-24.1176, 28.8875) (-24.1141, 28.8847) (-24.1107, 28.8819) (-24.1073, 28.8792) (-24.104, 28.8766) (-24.1008, 28.874) (-24.0976, 28.8714) (-24.0945, 28.8689) (-24.0914, 28.8665) (-24.0884, 28.8641) (-24.0855, 28.8618) (-24.0826, 28.8595) (-24.0798, 28.8573) (-24.077, 28.8551) (-24.0743, 28.853) (-24.0717, 28.851) (-24.0691, 28.849) (-24.0666, 28.8471) (-24.0641, 28.8452) (-24.0618, 28.8434) (-24.0595, 28.8416) (-24.0572, 28.8399) (-24.0551, 28.8383) (-24.053, 28.8367) (-24.051, 28.8352) (-24.049, 28.8338) (-24.0471, 28.8324) (-24.0453, 28.831) (-24.0436, 28.8298) (-24.042, 28.8286) (-24.0404, 28.8274) (-24.0389, 28.8263) (-24.0375, 28.8253) (-24.0362, 28.8244) (-24.035, 28.8235) (-24.0338, 28.8227) (-24.0327, 28.8219) (-24.0317, 28.8212) (-24.0309, 28.8206) (-24.0301, 28.82) (-24.0294, 28.8195) (-24.0287, 28.8191) (-24.0283, 28.8188) (-24.0281, 28.8186) (-24.0279, 28.8185) (-24.0278, 28.8184) knots -1 -1 -1 -1 -1 -1 -0.99583333 -0.99166667 -0.9875 -0.98333333 -0.97916667 -0.975 -0.97083333 -0.96666667 -0.9625 -0.95833333 -0.95416667 -0.95 -0.94583333 -0.94166667 -0.9375 -0.93333333 -0.92916667 -0.925 -0.92083333 -0.91666667 -0.9125 -0.90833333 -0.90416667 -0.9 -0.89583333 -0.89166667 -0.8875 -0.88333333 -0.87916667 -0.875 -0.87083333 -0.86666667 -0.8625 -0.85833333 -0.85416667 -0.85 -0.84583333 -0.84166667 -0.8375 -0.83333333 -0.82916667 -0.825 -0.82083333 -0.81666667 -0.8125 -0.80833333 -0.80416667 -0.8 -0.79583333 -0.79166667 -0.7875 -0.78333333 -0.77916667 -0.775 -0.77083333 -0.76666667 -0.7625 -0.75833333 -0.75416667 -0.75 -0.74583333 -0.74166667 -0.7375 -0.73333333 -0.72916667 -0.725 -0.72083333 -0.71666667 -0.7125 -0.70833333 -0.70416667 -0.7 -0.69583333 -0.69166667 -0.6875 -0.68333333 -0.67916667 -0.675 -0.67083333 -0.66666667 -0.6625 -0.65833333 -0.65416667 -0.65 -0.64583333 -0.64166667 -0.6375 -0.63333333 -0.62916667 -0.625 -0.62083333 -0.61666667 -0.6125 -0.60833333 -0.60416667 -0.6 -0.59583333 -0.59166667 -0.5875 -0.58333333 -0.57916667 -0.575 -0.57083333 -0.56666667 -0.5625 -0.55833333 -0.55416667 -0.55 -0.54583333 -0.54166667 -0.5375 -0.53333333 -0.52916667 -0.525 -0.52083333 -0.51666667 -0.5125 -0.50833333 -0.50416667 -0.5 -0.49583333 -0.49166667 -0.4875 -0.48333333 -0.47916667 -0.475 -0.47083333 -0.46666667 -0.4625 -0.45833333 -0.45416667 -0.45 -0.44583333 -0.44166667 -0.4375 -0.43333333 -0.42916667 -0.425 -0.42083333 -0.41666667 -0.4125 -0.40833333 -0.40416667 -0.4 -0.39583333 -0.39166667 -0.3875 -0.38333333 -0.37916667 -0.375 -0.37083333 -0.36666667 -0.3625 -0.35833333 -0.35416667 -0.35 -0.34583333 -0.34166667 -0.3375 -0.33333333 -0.32916667 -0.325 -0.32083333 -0.31666667 -0.3125 -0.30833333 -0.30416667 -0.3 -0.29583333 -0.29166667 -0.2875 -0.28333333 -0.27916667 -0.275 -0.27083333 -0.26666667 -0.2625 -0.25833333 -0.25416667 -0.25 -0.24583333 -0.24166667 -0.2375 -0.23333333 -0.22916667 -0.225 -0.22083333 -0.21666667 -0.2125 -0.20833333 -0.20416667 -0.2 -0.19583333 -0.19166667 -0.1875 -0.18333333 -0.17916667 -0.175 -0.17083333 -0.16666667 -0.1625 -0.15833333 -0.15416667 -0.15 -0.14583333 -0.14166667 -0.1375 -0.13333333 -0.12916667 -0.125 -0.12083333 -0.11666667 -0.1125 -0.10833333 -0.10416667 -0.1 -0.09583333 -0.09166667 -0.0875 -0.08333333 -0.07916667 -0.075 -0.07083333 -0.06666667 -0.0625 -0.05833333 -0.05416667 -0.05 -0.04583333 -0.04166667 -0.0375 -0.03333333 -0.02916667 -0.025 -0.02083333 -0.01666667 -0.0125 -0.00833333 -0.00416667 0 0 0 0 0 0
  arc A26 (-26.5997, 28.4204) -> (-27.0873, 27.5758) centre (0, 12.5) ccw
  line L60 (-0.9213, 41.5298) -> (-0.9119, 41.2355)
  line L61 (-3.9508, 41.2753) -> (-3.9507, 41.2745)
  line L62 (-17.8086, -10.4441) -> (-17.8091, -10.4448)
  spline S15 degree 5 poles (22.7084, 33.6029) (22.7059, 33.6018) (22.7009, 33.5998) (22.6934, 33.5967) (22.6834, 33.5925) (22.671, 33.5873) (22.6586, 33.5822) (22.6462, 33.577) (22.6339, 33.5718) (22.6217, 33.5666) (22.6094, 33.5614) (22.5972, 33.5562) (22.585, 33.551) (22.5729, 33.5458) (22.5608, 33.5406) (22.5487, 33.5354) (22.5367, 33.5302) (22.5247, 33.525) (22.5127, 33.5198) (22.5008, 33.5145) (22.4889, 33.5093) (22.4771, 33.5041) (22.4653, 33.4989) (22.4535, 33.4937) (22.4417, 33.4884) (22.43, 33.4832) (22.4184, 33.478) (22.4067, 33.4727) (22.3951, 33.4675) (22.3836, 33.4623) (22.3721, 33.457) (22.3606, 33.4518) (22.3491, 33.4466) (22.3377, 33.4413) (22.3264, 33.4361) (22.315, 33.4308) (22.3037, 33.4256) (22.2925, 33.4204) (22.2812, 33.4151) (22.2701, 33.4099) (22.2589, 33.4046) (22.2478, 33.3994) (22.2367, 33.3942) (22.2257, 33.3889) (22.2147, 33.3837) (22.2038, 33.3784) (22.1928, 33.3732) (22.182, 33.368) (22.1711, 33.3627) (22.1603, 33.3575) (22.1496, 33.3523) (22.1388, 33.347) (22.1281, 33.3418) (22.1175, 33.3366) (22.1069, 33.3313) (22.0963, 33.3261) (22.0858, 33.3209) (22.0753, 33.3157) (22.0649, 33.3105) (22.0544, 33.3052) (22.0441, 33.3) (22.0337, 33.2948) (22.0235, 33.2896) (22.0132, 33.2844) (22.003, 33.2792) (21.9928, 33.274) (21.9827, 33.2688) (21.9726, 33.2636) (21.9625, 33.2584) (21.9525, 33.2532) (21.9426, 33.248) (21.9326, 33.2429) (21.9228, 33.2377) (21.9129, 33.2325) (21.9031, 33.2274) (21.8933, 33.2222) (21.8836, 33.217) (21.8739, 33.2119) (21.8643, 33.2067) (21.8547, 33.2016) (21.8451, 33.1965) (21.8356, 33.1913) (21.8261, 33.1862) (21.8167, 33.1811) (21.8073, 33.176) (21.798, 33.1709) (21.7887, 33.1658) (21.7794, 33.1607) (21.7702, 33.1556) (21.761, 33.1505) (21.7519, 33.1454) (21.7428, 33.1404) (21.7337, 33.1353) (21.7247, 33.1303) (21.7158, 33.1252) (21.7068, 33.1202) (21.698, 33.1152) (21.6891, 33.1101) (21.6803, 33.1051) (21.6716, 33.1001) (21.6629, 33.0951) (21.6542, 33.0902) (21.6456, 33.0852) (21.6371, 33.0802) (21.6285, 33.0753) (21.6201, 33.0703) (21.6116, 33.0654) (21.6032, 33.0605) (21.5949, 33.0555) (21.5866, 33.0506) (21.5783, 33.0457) (21.5701, 33.0409) (21.5619, 33.036) (21.5538, 33.0311) (21.5458, 33.0263) (21.5377, 33.0214) (21.5297, 33.0166) (21.5218, 33.0118) (21.5139, 33.007) (21.5061, 33.0022) (21.4983, 32.9974) (21.4905, 32.9927) (21.4828, 32.9879) (21.4752, 32.9832) (21.4676, 32.9784) (21.46, 32.9737) (21.4525, 32.969) (21.445, 32.9644) (21.4376, 32.9597) (21.4302, 32.955) (21.4229, 32.9504) (21.4156, 32.9458) (21.4084, 32.9412) (21.4012, 32.9366) (21.3941, 32.932) (21.387, 32.9274) (21.38, 32.9229) (21.373, 32.9184) (21.3661, 32.9139) (21.3592, 32.9094) (21.3523, 32.9049) (21.3455, 32.9004) (21.3388, 32.896) (21.3321, 32.8916) (21.3255, 32.8872) (21.3189, 32.8828) (21.3124, 32.8784) (21.3059, 32.8741) (21.2995, 32.8698) (21.2931, 32.8655) (21.2867, 32.8612) (21.2805, 32.8569) (21.2742, 32.8527) (21.2681, 32.8484) (21.2619, 32.8442) (21.2559, 32.8401) (21.2498, 32.8359) (21.2439, 32.8318) (21.238, 32.8277) (21.2321, 32.8236) (21.2263, 32.8195) (21.2205, 32.8155) (21.2148, 32.8115) (21.2092, 32.8075) (21.2036, 32.8035) (21.1981, 32.7996) (21.1926, 32.7956) (21.1871, 32.7918) (21.1818, 32.7879) (21.1764, 32.7841) (21.1712, 32.7802) (21.166, 32.7765) (21.1608, 32.7727) (21.1557, 32.769) (21.1507, 32.7653) (21.1457, 32.7616) (21.1408, 32.758) (21.1359, 32.7544) (21.1311, 32.7508) (21.1263, 32.7472) (21.1216, 32.7437) (21.117, 32.7402) (21.1124, 32.7368) (21.1079, 32.7333) (21.1034, 32.73) (21.099, 32.7266) (21.0947, 32.7233) (21.0904, 32.72) (21.0862, 32.7167) (21.082, 32.7135) (21.0779, 32.7103) (21.0739, 32.7072) (21.0699, 32.7041) (21.066, 32.701) (21.0621, 32.698) (21.0583, 32.695) (21.0546, 32.692) (21.0509, 32.6891) (21.0473, 32.6862) (21.0437, 32.6834) (21.0403, 32.6806) (21.0368, 32.6778) (21.0335, 32.6751) (21.0302, 32.6724) (21.027, 32.6698) (21.0238, 32.6672) (21.0207, 32.6647) (21.0177, 32.6622) (21.0148, 32.6597) (21.0119, 32.6573) (21.009, 32.655) (21.0063, 32.6527) (21.0036, 32.6504) (21.001, 32.6482) (20.9984, 32.6461) (20.996, 32.644) (20.9936, 32.6419) (20.9912, 32.6399) (20.989, 32.638) (20.9868, 32.6361) (20.9847, 32.6343) (20.9826, 32.6325) (20.9806, 32.6308) (20.9787, 32.6291) (20.9769, 32.6275) (20.9752, 32.626) (20.9735, 32.6245) (20.9719, 32.623) (20.9704, 32.6217) (20.9689, 32.6204) (20.9675, 32.6192) (20.9663, 32.618) (20.9651, 32.6169) (20.9639, 32.6159) (20.9629, 32.6149) (20.9619, 32.614) (20.961, 32.6132) (20.9602, 32.6125) (20.9595, 32.6118) (20.9589, 32.6112) (20.9583, 32.6107) (20.958, 32.6104) (20.9577, 32.6102) (20.9576, 32.61) (20.9575, 32.61) knots -1 -1 -1 -1 -1 -1 -0.99583333 -0.99166667 -0.9875 -0.98333333 -0.97916667 -0.975 -0.97083333 -0.96666667 -0.9625 -0.95833333 -0.95416667 -0.95 -0.94583333 -0.94166667 -0.9375 -0.93333333 -0.92916667 -0.925 -0.92083333 -0.91666667 -0.9125 -0.90833333 -0.90416667 -0.9 -0.89583333 -0.89166667 -0.8875 -0.88333333 -0.87916667 -0.875 -0.87083333 -0.86666667 -0.8625 -0.85833333 -0.85416667 -0.85 -0.84583333 -0.84166667 -0.8375 -0.83333333 -0.82916667 -0.825 -0.82083333 -0.81666667 -0.8125 -0.80833333 -0.80416667 -0.8 -0.79583333 -0.79166667 -0.7875 -0.78333333 -0.77916667 -0.775 -0.77083333 -0.76666667 -0.7625 -0.75833333 -0.75416667 -0.75 -0.74583333 -0.74166667 -0.7375 -0.73333333 -0.72916667 -0.725 -0.72083333 -0.71666667 -0.7125 -0.70833333 -0.70416667 -0.7 -0.69583333 -0.69166667 -0.6875 -0.68333333 -0.67916667 -0.675 -0.67083333 -0.66666667 -0.6625 -0.65833333 -0.65416667 -0.65 -0.64583333 -0.64166667 -0.6375 -0.63333333 -0.62916667 -0.625 -0.62083333 -0.61666667 -0.6125 -0.60833333 -0.60416667 -0.6 -0.59583333 -0.59166667 -0.5875 -0.58333333 -0.57916667 -0.575 -0.57083333 -0.56666667 -0.5625 -0.55833333 -0.55416667 -0.55 -0.54583333 -0.54166667 -0.5375 -0.53333333 -0.52916667 -0.525 -0.52083333 -0.51666667 -0.5125 -0.50833333 -0.50416667 -0.5 -0.49583333 -0.49166667 -0.4875 -0.48333333 -0.47916667 -0.475 -0.47083333 -0.46666667 -0.4625 -0.45833333 -0.45416667 -0.45 -0.44583333 -0.44166667 -0.4375 -0.43333333 -0.42916667 -0.425 -0.42083333 -0.41666667 -0.4125 -0.40833333 -0.40416667 -0.4 -0.39583333 -0.39166667 -0.3875 -0.38333333 -0.37916667 -0.375 -0.37083333 -0.36666667 -0.3625 -0.35833333 -0.35416667 -0.35 -0.34583333 -0.34166667 -0.3375 -0.33333333 -0.32916667 -0.325 -0.32083333 -0.31666667 -0.3125 -0.30833333 -0.30416667 -0.3 -0.29583333 -0.29166667 -0.2875 -0.28333333 -0.27916667 -0.275 -0.27083333 -0.26666667 -0.2625 -0.25833333 -0.25416667 -0.25 -0.24583333 -0.24166667 -0.2375 -0.23333333 -0.22916667 -0.225 -0.22083333 -0.21666667 -0.2125 -0.20833333 -0.20416667 -0.2 -0.19583333 -0.19166667 -0.1875 -0.18333333 -0.17916667 -0.175 -0.17083333 -0.16666667 -0.1625 -0.15833333 -0.15416667 -0.15 -0.14583333 -0.14166667 -0.1375 -0.13333333 -0.12916667 -0.125 -0.12083333 -0.11666667 -0.1125 -0.10833333 -0.10416667 -0.1 -0.09583333 -0.09166667 -0.0875 -0.08333333 -0.07916667 -0.075 -0.07083333 -0.06666667 -0.0625 -0.05833333 -0.05416667 -0.05 -0.04583333 -0.04166667 -0.0375 -0.03333333 -0.02916667 -0.025 -0.02083333 -0.01666667 -0.0125 -0.00833333 -0.00416667 0 0 0 0 0 0